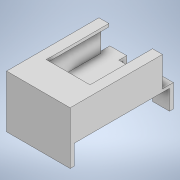
# Autodesk Inventor part: Camera_Mount
Saved by Autodesk Inventor 2021 (Build 250183000, 183)
## iProperties
Created: 2021-06-15
Part Number: Camera_Mount
Material: Generic
Document SubType Name: Modeling
Designer: Jorian Brusind
Density: 1 g/cm^3
Appearance: Default
Author: Jorian Brusind
Autodesk Inventor part; units mm, degrees
ref_plane "YZ Plane" through (0, 0, 0) normal (1, 0, 0) x (0, 1, 0)
ref_plane "XZ Plane" through (0, 0, 0) normal (0, 1, 0) x (-1, 0, 0)
ref_plane "XY Plane" through (0, 0, 0) normal (0, 0, 1) x (1, 0, 0)
sketch "Sketch1" plane through (0, 0, 0) normal (0, 1, 0) x (-1, 0, 0)
  line L0 (0, 0) -> (60, 0)
  line L1 (60, 0) -> (60, -84)
  line L2 (60, -84) -> (0, -84)
  line L3 (0, -84) -> (0, 0)
  line L4 (62, -86) -> (62, 2)
  line L5 (62, 2) -> (-2, 2)
  line L6 (-2, 2) -> (-2, -86)
  line L7 (-2, -86) -> (62, -86)
  dimension "d0" = 60
  dimension "d1" = 84
  dimension "d2" = 2
  constraints: 16 end point, 4 parallel, 2 perpendicular, 1 horizontal, 3 other
  measures "d0" distance of L1.end L2.end
  measures "d1" distance of L0.end L1.end
  measures "d2" distance between parallel lines of L1 L4
extrude "Extrusion1" add sketch "Sketch1" along normal blind 3 contours L0 L1 L2 L3 | L7 L6 L5 L4
sketch "Sketch2" plane through (0, 3, 0) normal (0, 1, 0) x (1, 0, 0)
  line L0 (0, 0) -> (-60, 0)
  line L1 (-60, 0) -> (-60, 84)
  line L2 (-60, 84) -> (0, 84)
  line L3 (0, 84) -> (0, 0)
  line L4 (2, 86) -> (-62, 86) projected
  line L5 (-62, -2) -> (2, -2) projected
  line L6 (-62, 86) -> (2, 86)
  line L7 (2, 86) -> (2, -2)
  line L8 (2, -2) -> (-62, -2)
  line L9 (-62, -2) -> (-62, 86)
  dimension "d5" = 60
  dimension "d6" = 84
  constraints: 16 end point, 4 parallel, 2 horizontal, 2 perpendicular
  measures "d5" distance of L1.end L2.end
  measures "d6" distance of L0.end L1.end
extrude "Extrusion2" add sketch "Sketch2" along normal blind 10
sketch "Sketch3" plane through (0, 0, 0) normal (0, -1, 0) x (1, 0, 0)
  circle A0 centre (-30.4, -71.4) radius 1.6
  circle A1 centre (-30.4, -11.4) radius 1.6
  circle A2 centre (-47.9, -41.4) radius 1.6
  circle A3 centre (-12.9, -41.4) radius 1.6
  line L0 (2, -86) -> (-62, -86) projected
  line L1 (-62, -86) -> (-62, 2) projected
  point P0 (0, 0)
  dimension "d9" = 3.2
  dimension "d10" = 3.2
  dimension "d11" = 3.2
  dimension "d12" = 3.2
  dimension "d13" = 60
  dimension "d14" = 35
  dimension "d15" = 17.5
  dimension "d16" = 30
  dimension "d17" = 30
  dimension "d18" = 17.5
  dimension "d19" = 14.6
  dimension "d20" = 14.1
  constraints: 4 centre point
  measures "d9" diameter of A0
  measures "d10" diameter of A1
  measures "d11" diameter of A2
  measures "d12" diameter of A3
  measures "d13" distance of A1.centre A0.centre
  measures "d14" distance of A3.centre A2.centre
  measures "d15" horizontal distance of A2.centre A0.centre
  measures "d16" vertical distance of A3.centre A0.centre
  measures "d17" vertical distance of A0.centre A2.centre
  measures "d18" horizontal distance of A1.centre A3.centre
  measures "d19" distance from line of L0 A0.centre
  measures "d20" distance from line of L1 A2.centre
extrude "Extrusion3" cut sketch "Sketch3" against normal through all
sketch "Sketch4" plane through (0, 13, 0) normal (0, 1, 0) x (1, 0, 0)
  line L0 (-60, 84) -> (0, 84) projected
  line L1 (0, 84) -> (-15, 84)
  line L2 (-60, 84) -> (-45, 84)
  line L3 (-45, 84) -> (-15, 84)
  line L4 (-15, 84) -> (-15, 86)
  line L5 (-15, 86) -> (-45, 86)
  line L6 (-45, 86) -> (-45, 84)
  point P0 (0, 0)
  dimension "d23" = 15
  dimension "d24" = 15
  dimension "d25" = 30
  dimension "d26" = 2
  constraints: 12 end point, 2 parallel, 2 point on line, 1 horizontal, 1 perpendicular
  measures "d23" distance of L0.end L1.end
  measures "d24" distance of L0.start L2.end
  measures "d25" distance of L5.end L4.end
  measures "d26" distance of L4.end L3.end
extrude "Extrusion4" cut sketch "Sketch4" against normal blind 10
sketch "Sketch5" plane through (0, 0, 0) normal (0, -1, 0) x (1, 0, 0)
  line L0 (2, -86) -> (-15, -86) projected
  line L1 (2, -86) -> (-62, -86)
  line L2 (-62, -86) -> (-62, -94)
  line L3 (-62, -94) -> (2, -94)
  line L4 (2, -94) -> (2, -86)
  line L5 (-62, 2) -> (2, 2) projected
  line L6 (2, 2) -> (-62, 2)
  line L7 (-62, 2) -> (-62, 10)
  line L8 (-62, 10) -> (2, 10)
  line L9 (2, 10) -> (2, 2)
  line L10 (-45, -86) -> (-15, -86) projected
  line L11 (-45, -86) -> (-15, -86)
  line L12 (-15, -86) -> (-15, -94)
  line L13 (-15, -94) -> (-45, -94)
  line L14 (-45, -94) -> (-45, -86)
  point P0 (0, 0)
  dimension "d29" = 64
  dimension "d30" = 8
  dimension "d31" = 64
  dimension "d32" = 8
  constraints: 24 end point, 6 parallel, 3 horizontal, 3 perpendicular, 1 point on line
  measures "d29" distance of L3.end L2.end
  measures "d30" distance of L2.end L1.end
  measures "d31" distance of L7.end L8.end
  measures "d32" distance of L6.end L7.end
extrude "Extrusion5" add sketch "Sketch5" against normal up to surface (13 mm away) contours L4 L3 L12 L0 | L14 L3 L2 L1 | L7 L8 L9 L5
sketch "Sketch6" plane through (0, 0, 0) normal (0, -1, 0) x (1, 0, 0)
  line L0 (2, 10) -> (-62, 10) projected
  line L1 (-62, 10) -> (2, 10)
  line L2 (2, 10) -> (2, 6)
  line L3 (2, 6) -> (-62, 6)
  line L4 (-62, 6) -> (-62, 10)
  line L5 (-62, 10) -> (-62, -94) projected
  line L6 (-62, 10) -> (-62, -94) projected
  line L7 (-62, -94) -> (-45, -94)
  line L8 (-45, -94) -> (-45, -90)
  line L9 (-45, -90) -> (-62, -90)
  line L10 (-62, -90) -> (-62, -94)
  line L11 (-15, -94) -> (2, -94) projected
  line L12 (2, -94) -> (-15, -94)
  line L13 (-15, -94) -> (-15, -90)
  line L14 (-15, -90) -> (2, -90)
  line L15 (2, -90) -> (2, -94)
  point P0 (0, 0)
  point P1 (-45, -86)
  point P2 (2, 10)
  dimension "d35" = 64
  dimension "d36" = 4
  dimension "d39" = 17
  dimension "d40" = 4
  dimension "d41" = 17
  dimension "d42" = 4
  constraints: 24 end point, 6 parallel, 3 horizontal, 3 perpendicular
  measures "d35" distance of L2.end L3.end
  measures "d36" distance of L1.end L2.end
  measures "d39" distance of L9.end L8.end
  measures "d40" distance of L8.end L7.end
  measures "d41" distance of L13.end L14.end
  measures "d42" distance of L12.end L13.end
extrude "Extrusion7" add sketch "Sketch6" along normal blind 20
move faces "Move1" translate (0, -10, 0) faces at (-40, 13, 6.6667)
sketch "Sketch8" plane through (-62, 3, 10) normal (0, 1, 0) x (1, 0, 0)
  line L0 (64, 0) -> (0, 0) projected
  line L1 (0, 0) -> (64, 0)
  line L2 (64, 0) -> (64, 95)
  line L3 (0, 95) -> (0, 0)
  line L4 (62, 93) -> (62, 2)
  line L5 (62, 2) -> (2, 2)
  line L6 (2, 2) -> (2, 93)
  line L7 (62, 93) -> (64, 93)
  line L8 (2, 93) -> (0, 93)
  line L9 (62, 2) -> (2, 2)
  line L10 (2, 2) -> (2, 10)
  line L11 (2, 10) -> (62, 10)
  line L12 (62, 10) -> (62, 2)
  point P0 (62, 10)
  point P1 (62, 10)
  dimension "d48" = 64
  dimension "d49" = 95
  dimension "d50" = 2
  dimension "d51" = 60
  dimension "d54" = 8
  constraints: 24 end point, 4 parallel, 4 point on line, 3 horizontal, 3 perpendicular, 2 other
  measures "d48" distance of L3.start L2.end
  measures "d49" distance of L2.end L1.end
  measures "d50" distance between parallel lines of L2 L4
  measures "d51" distance between parallel lines of L6 L4
  measures "d54" distance of L9.end L10.end
extrude "Extrusion9" add sketch "Sketch8" along normal blind 27
sketch "Sketch9" plane through (-62, 30, 10) normal (0, 1, 0) x (1, 0, 0)
  line L0 (62, 10) -> (62, 93) projected
  line L1 (62, 93) -> (54, 93)
  line L2 (54, 93) -> (54, 10)
  line L3 (54, 10) -> (62, 10)
  line L4 (62, 10) -> (62, 93)
  line L5 (2, 93) -> (2, 10) projected
  line L6 (2, 93) -> (10, 93)
  line L7 (10, 93) -> (10, 10)
  line L8 (10, 10) -> (2, 10)
  line L9 (2, 10) -> (2, 93)
  line L10 (2, 10) -> (62, 10) projected
  line L11 (62, 10) -> (2, 10)
  line L12 (2, 10) -> (2, 30)
  line L13 (2, 30) -> (62, 30)
  line L14 (62, 30) -> (62, 10)
  line L15 (64, 0) -> (64, 93) projected
  line L16 (64, 0) -> (0, 0)
  line L17 (0, 0) -> (0, 93)
  line L18 (0, 93) -> (64, 93)
  line L19 (64, 93) -> (64, 0)
  point P0 (54, 30)
  point P1 (10, 30)
  dimension "d57" = 8
  dimension "d58" = 8
  dimension "d59" = 83
  dimension "d60" = 60
  dimension "d61" = 20
  dimension "d62" = 64
  dimension "d63" = 93
  constraints: 32 end point, 8 parallel, 4 horizontal, 4 perpendicular
  measures "d57" distance of L3.end L2.end
  measures "d58" distance of L7.end L8.end
  measures "d59" distance of L6.end L7.end
  measures "d60" distance of L12.end L13.end
  measures "d61" distance of L11.end L12.end
  measures "d62" distance of L17.end L18.end
  measures "d63" distance of L16.end L17.end
extrude "Extrusion10" add sketch "Sketch9" along normal blind 3 contours L3 L2 L13 L0 | L0 L18 L15 L16 L17 L5 L8 L10 L3 | L13 L2 L1 L0 | L10 L7 L13 L2 | L8 L5 L13 L7 | L13 L5 L6 L7
body "Solid1"
